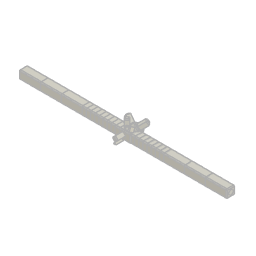
ModularFrame (Autodesk Fusion 360 design; units mm, degrees)
Autodesk Fusion 360 part; units mm, degrees
sketch "Sketch1" plane through (0, 0, 0) normal (0, 0, 1) x (1, 0, 0) in component "BasePart"
  line L0 (5, -5) -> (-5, -5)
  line L1 (-5, -5) -> (-5, 5)
  line L2 (-5, 5) -> (5, 5)
  line L3 (5, 5) -> (5, -5)
  line L4 (5, -5) -> (-5, 5) construction
  line L5 (-5, -5) -> (5, 5) construction
  dimension "drivingDimension" = 10
  constraint horizontal L0
  constraint perpendicular L0 L1
  constraint parallel L0 L2
  constraint parallel L1 L3
  constraint coincident L4 origin
  constraint coincident L5 origin
  constraint equal L1 L2
  measures "drivingDimension" distance of L1.end L2.end
extrude "Extrude1" add sketch "Sketch1" along normal blind 10 makes body 1 in component "BasePart"
chamfer "Chamfer1" distance 1 angle 45 6 faces at (5, 1.6667, 3.3333) (-1.6667, 1.6667, 10) (1.6667, -5, 3.3333) (-5, -1.6667, 3.3333) (-1.6667, 5, 3.3333) (-1.6667, 1.6667, 0) on bodies 1 in component "BasePart"
sketch "Sketch1 (2)" plane through (0, 0, 0) normal (0, 1, 0) x (1, 0, 0) in component "Peg"
  line L0 (0, -3.3333) -> (-3.3333, 0)
  line L1 (-3.3333, 0) -> (0, 3.3333)
  line L2 (0, 3.3333) -> (3.3333, 0)
  line L3 (3.3333, 0) -> (0, -3.3333)
  line L4 (0, 0) -> (3.3333, 0) construction
  line L5 (0, -3.3333) -> (0, 0) construction
  dimension "d266" = 3.3333
  dimension "d267" = 45
  constraint coincident L4.start L5.end
  constraint perpendicular L0 L1
  constraint parallel L0 L2
  constraint parallel L1 L3
  constraint horizontal L4
  constraint vertical L5
  constraint equal L0 L1
  measures "d266" distance of L4.start L2.end
  measures "d267" angle of L3 L4
extrude "Extrude1'" add sketch "Sketch1 (2)" along normal blind 10 separate body makes body 2 in component "Peg"
sketch "Sketch1 (3)" plane through (0, 0, 0) normal (0, 1, 0) x (1, 0, 0) in component "PegHoleCuttingTool"
  line L0 (0, -3.5333) -> (-3.5333, 0)
  line L1 (-3.5333, 0) -> (0, 3.5333)
  line L2 (0, 3.5333) -> (3.5333, 0)
  line L3 (3.5333, 0) -> (0, -3.5333)
  line L4 (0, -3.5333) -> (0, 0) construction
  line L5 (0, 0) -> (3.5333, 0) construction
  dimension "d268" = 3.5333
  dimension "d269" = 45
  constraint coincident L4.end L5.start
  constraint perpendicular L0 L1
  constraint parallel L0 L2
  constraint parallel L1 L3
  constraint vertical L4
  constraint perpendicular L4 L5
  constraint equal L0 L1
  measures "d268" distance of L4.end L2.end
  measures "d269" angle of L3 L5
extrude "Extrude1''" add sketch "Sketch1 (3)" along normal blind 10 separate body makes body 3 in component "PegHoleCuttingTool"
chamfer "Chamfer1'" distance 1 angle 45 1 faces at (0, 10, 1.1111) on bodies 2 in component "Peg"
sketch "Sketch1 (4)" plane through (0, 0, 0) normal (0, 0, 1) x (1, 0, 0) in component "Edge_2x"
  line L0 (10, 5) -> (-10, 5)
  line L1 (-10, 5) -> (-10, -5)
  line L2 (-10, -5) -> (10, -5)
  line L3 (10, -5) -> (10, 5)
  line L4 (10, 5) -> (-10, -5) construction
  line L5 (-10, 5) -> (10, -5) construction
  dimension "d165" = 20
  dimension "d166" = 10
  constraint horizontal L0
  constraint perpendicular L0 L1
  constraint parallel L0 L2
  constraint parallel L1 L3
  constraint coincident L4 origin
  constraint coincident L5 origin
  measures "d165" distance of L1.end L2.end
  measures "d166" distance of L0.end L1.end
extrude "Extrude1'''" add sketch "Sketch1 (4)" along normal blind 10 separate body makes body 4 in component "Edge_2x"
chamfer "Chamfer1''" distance 1 angle 45 6 faces at (-3.3333, -5, 3.3333) (-3.3333, 1.6667, 10) (-10, 1.6667, 3.3333) (3.3333, 5, 3.3333) (10, -1.6667, 3.3333) (-3.3333, 1.6667, 0) on bodies 4 in component "Edge_2x"
combine "Combine1" operation cut target body 4 tool bodies 3 3 body 3 seen with x (0, -1, 0) y (-1, 0, 0) z (0, 0, -1) at (0, 0, 5) body 3 seen with x (0, 1, 0) y (1, 0, 0) z (0, 0, -1) at (0, 0, 5) keep tools in component "Edge_2x"
sketch "Sketch1 (5)" plane through (0, 0, 0) normal (0, 0, 1) x (1, 0, 0) in component "Edge_3x"
  line L0 (15, 5) -> (-15, 5)
  line L1 (-15, 5) -> (-15, -5)
  line L2 (-15, -5) -> (15, -5)
  line L3 (15, -5) -> (15, 5)
  line L4 (15, 5) -> (-15, -5) construction
  line L5 (-15, 5) -> (15, -5) construction
  dimension "d165_1" = 30
  dimension "d166_1" = 10
  constraint horizontal L0
  constraint perpendicular L0 L1
  constraint parallel L0 L2
  constraint parallel L1 L3
  constraint coincident L4 origin
  constraint coincident L5 origin
  measures "d165_1" distance of L1.end L2.end
  measures "d166_1" distance of L0.end L1.end
extrude "Extrude1''''" add sketch "Sketch1 (5)" along normal blind 10 separate body makes body 5 in component "Edge_3x"
chamfer "Chamfer1'''" distance 1 angle 45 6 faces at (-5, -5, 3.3333) (-5, -1.6667, 10) (-15, 1.6667, 3.3333) (5, 5, 3.3333) (15, -1.6667, 3.3333) (-5, -1.6667, 0) on bodies 5 in component "Edge_3x"
sketch "Sketch1 (6)" plane through (0, 0, 0) normal (0, 0, 1) x (1, 0, 0) in component "Edge_4x"
  line L0 (20, 5) -> (-20, 5)
  line L1 (-20, 5) -> (-20, -5)
  line L2 (-20, -5) -> (20, -5)
  line L3 (20, -5) -> (20, 5)
  line L4 (20, 5) -> (-20, -5) construction
  line L5 (-20, 5) -> (20, -5) construction
  dimension "d165_1_1" = 40
  dimension "d166_1_1" = 10
  constraint horizontal L0
  constraint perpendicular L0 L1
  constraint parallel L0 L2
  constraint parallel L1 L3
  constraint coincident L4 origin
  constraint coincident L5 origin
  measures "d165_1_1" distance of L1.end L2.end
  measures "d166_1_1" distance of L0.end L1.end
extrude "Extrude1'''''" add sketch "Sketch1 (6)" along normal blind 10 separate body makes body 6 in component "Edge_4x"
chamfer "Chamfer1''''" distance 1 angle 45 6 faces at (-6.6667, -5, 3.3333) (-6.6667, 1.6667, 10) (-20, 1.6667, 3.3333) (6.6667, 5, 3.3333) (20, -1.6667, 3.3333) (-6.6667, 1.6667, 0) on bodies 6 in component "Edge_4x"
sketch "Sketch1 (7)" plane through (0, 0, 0) normal (0, 0, 1) x (1, 0, 0) in component "Edge_5x"
  line L0 (25, 5) -> (-25, 5)
  line L1 (-25, 5) -> (-25, -5)
  line L2 (-25, -5) -> (25, -5)
  line L3 (25, -5) -> (25, 5)
  line L4 (25, 5) -> (-25, -5) construction
  line L5 (-25, 5) -> (25, -5) construction
  dimension "d165_1_2" = 50
  dimension "d166_1_2" = 10
  constraint horizontal L0
  constraint perpendicular L0 L1
  constraint parallel L0 L2
  constraint parallel L1 L3
  constraint coincident L4 origin
  constraint coincident L5 origin
  measures "d165_1_2" distance of L1.end L2.end
  measures "d166_1_2" distance of L0.end L1.end
extrude "Extrude1''''''" add sketch "Sketch1 (7)" along normal blind 10 separate body makes body 7 in component "Edge_5x"
chamfer "Chamfer1'''''" distance 1 angle 45 6 faces at (-8.3333, -5, 3.3333) (-8.3333, 1.6667, 10) (-25, 1.6667, 3.3333) (8.3333, 5, 3.3333) (25, -1.6667, 3.3333) (-8.3333, 1.6667, 0) on bodies 7 in component "Edge_5x"
sketch "Sketch1 (8)" plane through (0, 0, 0) normal (0, 0, 1) x (1, 0, 0) in component "Edge_6x"
  line L0 (30, 5) -> (-30, 5)
  line L1 (-30, 5) -> (-30, -5)
  line L2 (-30, -5) -> (30, -5)
  line L3 (30, -5) -> (30, 5)
  line L4 (30, 5) -> (-30, -5) construction
  line L5 (-30, 5) -> (30, -5) construction
  dimension "d165_1_3" = 60
  dimension "d166_1_3" = 10
  constraint horizontal L0
  constraint perpendicular L0 L1
  constraint parallel L0 L2
  constraint parallel L1 L3
  constraint coincident L4 origin
  constraint coincident L5 origin
  measures "d165_1_3" distance of L1.end L2.end
  measures "d166_1_3" distance of L0.end L1.end
extrude "Extrude1'''''''" add sketch "Sketch1 (8)" along normal blind 10 separate body makes body 8 in component "Edge_6x"
chamfer "Chamfer1''''''" distance 1 angle 45 6 faces at (-10, -5, 3.3333) (-10, 1.6667, 10) (-30, 1.6667, 3.3333) (10, 5, 3.3333) (30, -1.6667, 3.3333) (-10, 1.6667, 0) on bodies 8 in component "Edge_6x"
sketch "Sketch1 (9)" plane through (0, 0, 0) normal (0, 0, 1) x (1, 0, 0) in component "Edge_7x"
  line L0 (35, 5) -> (-35, 5)
  line L1 (-35, 5) -> (-35, -5)
  line L2 (-35, -5) -> (35, -5)
  line L3 (35, -5) -> (35, 5)
  line L4 (35, 5) -> (-35, -5) construction
  line L5 (-35, 5) -> (35, -5) construction
  dimension "d165_1_4" = 70
  dimension "d166_1_4" = 10
  constraint horizontal L0
  constraint perpendicular L0 L1
  constraint parallel L0 L2
  constraint parallel L1 L3
  constraint coincident L4 origin
  constraint coincident L5 origin
  measures "d165_1_4" distance of L1.end L2.end
  measures "d166_1_4" distance of L0.end L1.end
extrude "Extrude1''''''''" add sketch "Sketch1 (9)" along normal blind 10 separate body makes body 9 in component "Edge_7x"
chamfer "Chamfer1'''''''" distance 1 angle 45 6 faces at (-11.6667, -5, 3.3333) (-11.6667, 1.6667, 10) (-35, 1.6667, 3.3333) (11.6667, 5, 3.3333) (35, -1.6667, 3.3333) (-11.6667, 1.6667, 0) on bodies 9 in component "Edge_7x"
sketch "Sketch1 (10)" plane through (0, 0, 0) normal (0, 0, 1) x (1, 0, 0) in component "Edge_8x"
  line L0 (40, 5) -> (-40, 5)
  line L1 (-40, 5) -> (-40, -5)
  line L2 (-40, -5) -> (40, -5)
  line L3 (40, -5) -> (40, 5)
  line L4 (40, 5) -> (-40, -5) construction
  line L5 (-40, 5) -> (40, -5) construction
  dimension "d165_1_5" = 80
  dimension "d166_1_5" = 10
  constraint horizontal L0
  constraint perpendicular L0 L1
  constraint parallel L0 L2
  constraint parallel L1 L3
  constraint coincident L4 origin
  constraint coincident L5 origin
  measures "d165_1_5" distance of L1.end L2.end
  measures "d166_1_5" distance of L0.end L1.end
extrude "Extrude1'''''''''" add sketch "Sketch1 (10)" along normal blind 10 separate body makes body 10 in component "Edge_8x"
chamfer "Chamfer1''''''''" distance 1 angle 45 6 faces at (-13.3333, -5, 6.6667) (13.3333, 1.6667, 10) (-40, 1.6667, 3.3333) (13.3333, 5, 6.6667) (40, -1.6667, 3.3333) (13.3333, 1.6667, 0) on bodies 10 in component "Edge_8x"
sketch "Sketch1 (11)" plane through (0, 0, 0) normal (0, 0, 1) x (1, 0, 0) in component "Edge_9x"
  line L0 (45, 5) -> (-45, 5)
  line L1 (-45, 5) -> (-45, -5)
  line L2 (-45, -5) -> (45, -5)
  line L3 (45, -5) -> (45, 5)
  line L4 (45, 5) -> (-45, -5) construction
  line L5 (-45, 5) -> (45, -5) construction
  dimension "d165_1_6" = 90
  dimension "d166_1_6" = 10
  constraint horizontal L0
  constraint perpendicular L0 L1
  constraint parallel L0 L2
  constraint parallel L1 L3
  constraint coincident L4 origin
  constraint coincident L5 origin
  measures "d165_1_6" distance of L1.end L2.end
  measures "d166_1_6" distance of L0.end L1.end
extrude "Extrude1''''''''''" add sketch "Sketch1 (11)" along normal blind 10 separate body makes body 11 in component "Edge_9x"
chamfer "Chamfer1'''''''''" distance 1 angle 45 6 faces at (-15, -5, 3.3333) (15, -1.6667, 10) (-45, 1.6667, 3.3333) (15, 5, 3.3333) (45, -1.6667, 3.3333) (15, -1.6667, 0) on bodies 11 in component "Edge_9x"
sketch "Sketch1 (12)" plane through (0, 0, 0) normal (0, 0, 1) x (1, 0, 0) in component "Edge_10x"
  line L0 (50, 5) -> (-50, 5)
  line L1 (-50, 5) -> (-50, -5)
  line L2 (-50, -5) -> (50, -5)
  line L3 (50, -5) -> (50, 5)
  line L4 (50, 5) -> (-50, -5) construction
  line L5 (-50, 5) -> (50, -5) construction
  dimension "d165_1_7" = 100
  dimension "d166_1_7" = 10
  constraint horizontal L0
  constraint perpendicular L0 L1
  constraint parallel L0 L2
  constraint parallel L1 L3
  constraint coincident L4 origin
  constraint coincident L5 origin
  measures "d165_1_7" distance of L1.end L2.end
  measures "d166_1_7" distance of L0.end L1.end
extrude "Extrude1'''''''''''" add sketch "Sketch1 (12)" along normal blind 10 separate body makes body 12 in component "Edge_10x"
chamfer "Chamfer1''''''''''" distance 1 angle 45 6 faces at (-16.6667, -5, 3.3333) (16.6667, -1.6667, 10) (-50, 1.6667, 3.3333) (16.6667, 5, 3.3333) (50, -1.6667, 3.3333) (16.6667, -1.6667, 0) on bodies 12 in component "Edge_10x"
sketch "Sketch1 (13)" plane through (0, 0, 0) normal (0, 0, 1) x (1, 0, 0) in component "Edge_15x"
  line L0 (75, 5) -> (-75, 5)
  line L1 (-75, 5) -> (-75, -5)
  line L2 (-75, -5) -> (75, -5)
  line L3 (75, -5) -> (75, 5)
  line L4 (75, 5) -> (-75, -5) construction
  line L5 (-75, 5) -> (75, -5) construction
  dimension "d165_1_8" = 150
  dimension "d166_1_8" = 10
  constraint horizontal L0
  constraint perpendicular L0 L1
  constraint parallel L0 L2
  constraint parallel L1 L3
  constraint coincident L4 origin
  constraint coincident L5 origin
  measures "d165_1_8" distance of L1.end L2.end
  measures "d166_1_8" distance of L0.end L1.end
extrude "Extrude1''''''''''''" add sketch "Sketch1 (13)" along normal blind 10 separate body makes body 13 in component "Edge_15x"
chamfer "Chamfer1'''''''''''" distance 1 angle 45 6 faces at (-25, -5, 6.6667) (25, -1.6667, 10) (-75, 1.6667, 3.3333) (25, 5, 3.3333) (75, -1.6667, 3.3333) (25, -1.6667, 0) on bodies 13 in component "Edge_15x"
sketch "Sketch1 (14)" plane through (0, 0, 0) normal (0, 0, 1) x (1, 0, 0) in component "Edge_20x"
  line L0 (100, 5) -> (-100, 5)
  line L1 (-100, 5) -> (-100, -5)
  line L2 (-100, -5) -> (100, -5)
  line L3 (100, -5) -> (100, 5)
  line L4 (100, 5) -> (-100, -5) construction
  line L5 (-100, 5) -> (100, -5) construction
  dimension "d165_1_8_1" = 200
  dimension "d166_1_8_1" = 10
  constraint horizontal L0
  constraint perpendicular L0 L1
  constraint parallel L0 L2
  constraint parallel L1 L3
  constraint coincident L4 origin
  constraint coincident L5 origin
  measures "d165_1_8_1" distance of L1.end L2.end
  measures "d166_1_8_1" distance of L0.end L1.end
extrude "Extrude1'''''''''''''" add sketch "Sketch1 (14)" along normal blind 10 separate body makes body 14 in component "Edge_20x"
chamfer "Chamfer1''''''''''''" distance 1 angle 45 6 faces at (-33.3333, -5, 3.3333) (33.3333, 1.6667, 10) (-100, 1.6667, 3.3333) (33.3333, 5, 3.3333) (100, -1.6667, 3.3333) (33.3333, 1.6667, 0) on bodies 14 in component "Edge_20x"
sketch "Sketch1 (15)" plane through (0, 0, 0) normal (0, 0, 1) x (1, 0, 0) in component "Edge_25x"
  line L0 (125, 5) -> (-125, 5)
  line L1 (-125, 5) -> (-125, -5)
  line L2 (-125, -5) -> (125, -5)
  line L3 (125, -5) -> (125, 5)
  line L4 (125, 5) -> (-125, -5) construction
  line L5 (-125, 5) -> (125, -5) construction
  dimension "d165_1_8_2" = 250
  dimension "d166_1_8_2" = 10
  constraint horizontal L0
  constraint perpendicular L0 L1
  constraint parallel L0 L2
  constraint parallel L1 L3
  constraint coincident L4 origin
  constraint coincident L5 origin
  measures "d165_1_8_2" distance of L1.end L2.end
  measures "d166_1_8_2" distance of L0.end L1.end
extrude "Extrude1''''''''''''''" add sketch "Sketch1 (15)" along normal blind 10 separate body makes body 15 in component "Edge_25x"
chamfer "Chamfer1'''''''''''''" distance 1 angle 45 6 faces at (-41.6667, -5, 3.3333) (41.6667, -1.6667, 10) (-125, 1.6667, 3.3333) (41.6667, 5, 3.3333) (125, -1.6667, 3.3333) (41.6667, -1.6667, 0) on bodies 15 in component "Edge_25x"
combine "Combine2" operation cut target body 5 tool bodies 3 3 body 3 seen with x (0, 1, 0) y (-1, 0, 0) z (0, 0, 1) at (15, 0, 5) body 3 seen with x (0, -1, 0) y (1, 0, 0) z (0, 0, 1) at (-15, 0, 5) keep tools in component "Edge_3x"
combine "Combine2'" operation cut target body 6 tool bodies 3 3 body 3 seen with x (0, 1, 0) y (-1, 0, 0) z (0, 0, 1) at (20, 0, 5) body 3 seen with x (0, 0, 1) y (1, 0, 0) z (0, 1, 0) at (-20, 0, 5) keep tools in component "Edge_4x"
combine "Combine2''" operation cut target body 7 tool bodies 3 3 body 3 seen with x (0, 1, 0) y (-1, 0, 0) z (0, 0, 1) at (25, 0, 5) body 3 seen with x (0, -1, 0) y (1, 0, 0) z (0, 0, 1) at (-25, 0, 5) keep tools in component "Edge_5x"
combine "Combine2'''" operation cut target body 8 tool bodies 3 3 body 3 seen with x (0, 1, 0) y (-1, 0, 0) z (0, 0, 1) at (30, 0, 5) body 3 seen with x (0, -1, 0) y (1, 0, 0) z (0, 0, 1) at (-30, 0, 5) keep tools in component "Edge_6x"
combine "Combine2''''" operation cut target body 9 tool bodies 3 3 body 3 seen with x (0, -1, 0) y (1, 0, 0) z (0, 0, 1) at (-35, 0, 5) body 3 seen with x (0, 1, 0) y (-1, 0, 0) z (0, 0, 1) at (35, 0, 5) keep tools in component "Edge_7x"
combine "Combine2'''''" operation cut target body 10 tool bodies 3 3 body 3 seen with x (0, -1, 0) y (1, 0, 0) z (0, 0, 1) at (-40, 0, 5) body 3 seen with x (0, 1, 0) y (-1, 0, 0) z (0, 0, 1) at (40, 0, 5) keep tools in component "Edge_8x"
combine "Combine2''''''" operation cut target body 11 tool bodies 3 3 body 3 seen with x (0, 1, 0) y (-1, 0, 0) z (0, 0, 1) at (45, 0, 5) body 3 seen with x (0, -1, 0) y (1, 0, 0) z (0, 0, 1) at (-45, 0, 5) keep tools in component "Edge_9x"
combine "Combine2'''''''" operation cut target body 12 tool bodies 3 3 body 3 seen with x (0, 1, 0) y (-1, 0, 0) z (0, 0, 1) at (50, 0, 5) body 3 seen with x (0, -1, 0) y (1, 0, 0) z (0, 0, 1) at (-50, 0, 5) keep tools in component "Edge_10x"
combine "Combine2''''''''" operation cut target body 13 tool bodies 3 3 body 3 seen with x (0, -1, 0) y (1, 0, 0) z (0, 0, 1) at (-75, 0, 5) body 3 seen with x (0, 1, 0) y (-1, 0, 0) z (0, 0, 1) at (75, 0, 5) keep tools in component "Edge_15x"
combine "Combine2'''''''''" operation cut target body 14 tool bodies 3 3 body 3 seen with x (0, 1, 0) y (-1, 0, 0) z (0, 0, 1) at (100, 0, 5) body 3 seen with x (0, -1, 0) y (1, 0, 0) z (0, 0, 1) at (-100, 0, 5) keep tools in component "Edge_20x"
combine "Combine2''''''''''" operation cut target body 15 tool bodies 3 3 body 3 seen with x (0, 1, 0) y (-1, 0, 0) z (0, 0, 1) at (125, 0, 5) body 3 seen with x (0, -1, 0) y (1, 0, 0) z (0, 0, 1) at (-125, 0, 5) keep tools in component "Edge_25x"
sketch "Sketch1 (16)" plane through (0, 0, 0) normal (1, 0, 0) x (0, 1, 0) in component "Support"
  line L0 (0, 0) -> (3.3333, 0)
  line L1 (1.6667, 0) -> (1.6667, 1.6667) construction
  line L2 (1.6667, 1.6667) -> (3.3333, 0)
  line L3 (0, 0) -> (1.6667, 1.6667)
  dimension "d272" = 3.3333
  dimension "d273" = 1.6667
  constraint coincident L0.start L3.start
  constraint horizontal L0
  constraint midpoint L0 L1.start
  constraint perpendicular L0 L1
  measures "d272" distance of L0.start L0.end
  measures "d273" distance of L1.start L1.end
extrude "Extrude1'''''''''''''''" add sketch "Sketch1 (16)" along normal blind 9 separate body makes body 16 in component "Support"
combine "Combine1'" operation add target body 1 tool bodies 2 2 2 2 2 2 body 2 seen with x (0, 1, 0) y (-1, 0, 0) z (0, 0, 1) at (-5, 0, 5) body 2 seen with x (1, 0, 0) y (0, 0, 1) z (0, -1, 0) at (0, 0, 10) body 2 seen with x (1, 0, 0) y (0, 0, -1) z (0, 1, 0) at (0, 0, 0) body 2 seen with x (1, 0, 0) y (0, -1, 0) z (0, 0, -1) at (0, -5, 5) body 2 seen with x (1, 0, 0) y (0, 1, 0) z (0, 0, 1) at (0, 5, 5) body 2 seen with x (0, -1, 0) y (1, 0, 0) z (0, 0, 1) at (5, 0, 5) keep tools result as body 17 in component "AsNewCombinedComponent"
move_body "Align2" bodies 17 to x (0.788675, -0.211325, -0.57735) y (-0.211325, 0.788675, -0.57735) z (0.57735, 0.57735, 0.57735) at (1.4161, 1.4161, 4.6188) in component "AsNewCombinedComponent"
move_body "Move2" bodies 4 to x (1, 0, 0) y (0, 1, 0) z (0, 0, 1) at (170, -150, 0) in component "Edge_2x"
component "BasePart" placed x (1, 0, 0) y (0, 1, 0) z (0, 0, 1) at (0, 0, 0)
component "Peg" placed x (1, 0, 0) y (0, 1, 0) z (0, 0, 1) at (0, 0, 0)
component "PegHoleCuttingTool" placed x (1, 0, 0) y (0, 1, 0) z (0, 0, 1) at (0, 0, 0)
component "Support" placed x (0, -1, 0) y (1, 0, 0) z (0, 0, 1) at (-1.6667, -5, 0)
component "Connector_Extender" placed x (1, 0, 0) y (0, 1, 0) z (0, 0, 1) at (0, 0, 0)
component "Connector_3-sided_flat" placed x (1, 0, 0) y (0, 1, 0) z (0, 0, 1) at (0, 0, 0)
component "Connector_3-sided_corner" placed x (1, 0, 0) y (0, 1, 0) z (0, 0, 1) at (0, 0, 0)
component "Connector_4-sided_flat" placed x (1, 0, 0) y (0, 1, 0) z (0, 0, 1) at (0, 0, 0)
component "Connector_4-sided_corner" placed x (1, 0, 0) y (0, 1, 0) z (0, 0, 1) at (0, 0, 0)
component "Connector_5-sided" placed x (1, 0, 0) y (0, 1, 0) z (0, 0, 1) at (0, 0, 0)
component "Connector_6-sided" placed x (1, 0, 0) y (0, 1, 0) z (0, 0, 1) at (0, 0, 0)
component "Edge_2x" placed x (1, 0, 0) y (0, 1, 0) z (0, 0, 1) at (0, 0, 0)
component "Edge_3x" placed x (1, 0, 0) y (0, 1, 0) z (0, 0, 1) at (0, 0, 0)
component "Edge_4x" placed x (1, 0, 0) y (0, 1, 0) z (0, 0, 1) at (0, 0, 0)
component "Edge_5x" placed x (1, 0, 0) y (0, 1, 0) z (0, 0, 1) at (0, 0, 0)
component "Edge_6x" placed x (1, 0, 0) y (0, 1, 0) z (0, 0, 1) at (0, 0, 0)
component "Edge_7x" placed x (1, 0, 0) y (0, 1, 0) z (0, 0, 1) at (0, 0, 0)
component "Edge_8x" placed x (1, 0, 0) y (0, 1, 0) z (0, 0, 1) at (0, 0, 0)
component "Edge_9x" placed x (1, 0, 0) y (0, 1, 0) z (0, 0, 1) at (0, 0, 0)
component "Edge_10x" placed x (1, 0, 0) y (0, 1, 0) z (0, 0, 1) at (0, 0, 0)
component "Edge_15x" placed x (1, 0, 0) y (0, 1, 0) z (0, 0, 1) at (0, 0, 0)
component "Edge_20x" placed x (1, 0, 0) y (0, 1, 0) z (0, 0, 1) at (0, 0, 0)
component "Edge_25x" placed x (1, 0, 0) y (0, 1, 0) z (0, 0, 1) at (0, 0, 0)
component "ElementsShowcase" placed x (1, 0, 0) y (0, 1, 0) z (0, 0, 1) at (0, 0, 0)
component "BasePart" placed x (1, 0, 0) y (0, 1, 0) z (0, 0, 1) at (0, 0, 0) in component "Connector_Extender"
component "Peg" placed x (1, 0, 0) y (0, 1, 0) z (0, 0, 1) at (0, 5, 5) in component "Connector_Extender"
component "Peg" placed x (1, 0, 0) y (0, -1, 0) z (0, 0, -1) at (0, -5, 5) in component "Connector_Extender"
component "Support" placed x (0, 1, 0) y (-1, 0, 0) z (0, 0, 1) at (1.6667, 6, 0) in component "Connector_Extender"
component "Support" placed x (0, -1, 0) y (1, 0, 0) z (0, 0, 1) at (-1.6667, -6, 0) in component "Connector_Extender"
component "BasePart" placed x (1, 0, 0) y (0, 1, 0) z (0, 0, 1) at (0, 0, 0) in component "Connector_3-sided_flat"
component "Peg" placed x (1, 0, 0) y (0, 1, 0) z (0, 0, 1) at (0, 5, 5) in component "Connector_3-sided_flat"
component "Peg" placed x (0, -1, 0) y (1, 0, 0) z (0, 0, 1) at (5, 0, 5) in component "Connector_3-sided_flat"
component "Peg" placed x (1, 0, 0) y (0, -1, 0) z (0, 0, -1) at (0, -5, 5) in component "Connector_3-sided_flat"
component "Support" placed x (0, -1, 0) y (1, 0, 0) z (0, 0, 1) at (-1.6667, -6, 0) in component "Connector_3-sided_flat"
component "Support" placed x (0, 1, 0) y (-1, 0, 0) z (0, 0, 1) at (1.6667, 6, 0) in component "Connector_3-sided_flat"
component "Support" placed x (1, 0, 0) y (0, 1, 0) z (0, 0, 1) at (6, -1.6667, 0) in component "Connector_3-sided_flat"
component "BasePart" placed x (1, 0, 0) y (0, 1, 0) z (0, 0, 1) at (0, 0, 0) in component "Connector_3-sided_corner"
component "Peg" placed x (1, 0, 0) y (0, -1, 0) z (0, 0, -1) at (0, -5, 5) in component "Connector_3-sided_corner"
component "Peg" placed x (1, 0, 0) y (0, 0, 1) z (0, -1, 0) at (0, 0, 10) in component "Connector_3-sided_corner"
component "Peg" placed x (0, -1, 0) y (1, 0, 0) z (0, 0, 1) at (5, 0, 5) in component "Connector_3-sided_corner"
component "Support" placed x (0, -1, 0) y (1, 0, 0) z (0, 0, 1) at (-1.6667, -6, 0) in component "Connector_3-sided_corner"
component "Support" placed x (1, 0, 0) y (0, 1, 0) z (0, 0, 1) at (6, -1.6667, 0) in component "Connector_3-sided_corner"
component "BasePart" placed x (1, 0, 0) y (0, 1, 0) z (0, 0, 1) at (0, 0, 0) in component "Connector_4-sided_flat"
component "Peg" placed x (1, 0, 0) y (0, 1, 0) z (0, 0, 1) at (0, 5, 5) in component "Connector_4-sided_flat"
component "Peg" placed x (0, 1, 0) y (-1, 0, 0) z (0, 0, 1) at (-5, 0, 5) in component "Connector_4-sided_flat"
component "Peg" placed x (0, -1, 0) y (1, 0, 0) z (0, 0, 1) at (5, 0, 5) in component "Connector_4-sided_flat"
component "Peg" placed x (1, 0, 0) y (0, -1, 0) z (0, 0, -1) at (0, -5, 5) in component "Connector_4-sided_flat"
component "Support" placed x (0, -1, 0) y (1, 0, 0) z (0, 0, 1) at (-1.6667, -6, 0) in component "Connector_4-sided_flat"
component "Support" placed x (-1, 0, 0) y (0, -1, 0) z (0, 0, 1) at (-6, 1.6667, 0) in component "Connector_4-sided_flat"
component "Support" placed x (1, 0, 0) y (0, 1, 0) z (0, 0, 1) at (6, -1.6667, 0) in component "Connector_4-sided_flat"
component "Support" placed x (0, 1, 0) y (-1, 0, 0) z (0, 0, 1) at (1.6667, 6, 0) in component "Connector_4-sided_flat"
component "BasePart" placed x (1, 0, 0) y (0, 1, 0) z (0, 0, 1) at (0, 0, 0) in component "Connector_4-sided_corner"
component "Peg" placed x (0, -1, 0) y (1, 0, 0) z (0, 0, 1) at (5, 0, 5) in component "Connector_4-sided_corner"
component "Peg" placed x (1, 0, 0) y (0, 0, 1) z (0, -1, 0) at (0, 0, 10) in component "Connector_4-sided_corner"
component "Peg" placed x (1, 0, 0) y (0, 1, 0) z (0, 0, 1) at (0, 5, 5) in component "Connector_4-sided_corner"
component "Peg" placed x (1, 0, 0) y (0, -1, 0) z (0, 0, -1) at (0, -5, 5) in component "Connector_4-sided_corner"
component "Support" placed x (0, 1, 0) y (-1, 0, 0) z (0, 0, 1) at (1.6667, 6, 0) in component "Connector_4-sided_corner"
component "Support" placed x (1, 0, 0) y (0, 1, 0) z (0, 0, 1) at (6, -1.6667, 0) in component "Connector_4-sided_corner"
component "Support" placed x (0, -1, 0) y (1, 0, 0) z (0, 0, 1) at (-1.6667, -6, 0) in component "Connector_4-sided_corner"
component "BasePart" placed x (1, 0, 0) y (0, 1, 0) z (0, 0, 1) at (0, 0, 0) in component "Connector_5-sided"
component "Peg" placed x (1, 0, 0) y (0, -1, 0) z (0, 0, -1) at (0, -5, 5) in component "Connector_5-sided"
component "Peg" placed x (0, 1, 0) y (-1, 0, 0) z (0, 0, 1) at (-5, 0, 5) in component "Connector_5-sided"
component "Peg" placed x (1, 0, 0) y (0, 0, 1) z (0, -1, 0) at (0, 0, 10) in component "Connector_5-sided"
component "Peg" placed x (1, 0, 0) y (0, 1, 0) z (0, 0, 1) at (0, 5, 5) in component "Connector_5-sided"
component "Peg" placed x (0, -1, 0) y (1, 0, 0) z (0, 0, 1) at (5, 0, 5) in component "Connector_5-sided"
component "Support" placed x (1, 0, 0) y (0, 1, 0) z (0, 0, 1) at (6, -1.6667, 0) in component "Connector_5-sided"
component "Support" placed x (0, -1, 0) y (1, 0, 0) z (0, 0, 1) at (-1.6667, -6, 0) in component "Connector_5-sided"
component "Support" placed x (0, 1, 0) y (-1, 0, 0) z (0, 0, 1) at (1.6667, 6, 0) in component "Connector_5-sided"
component "Support" placed x (-1, 0, 0) y (0, -1, 0) z (0, 0, 1) at (-6, 1.6667, 0) in component "Connector_5-sided"
component "BasePart" placed x (1, 0, 0) y (0, 1, 0) z (0, 0, 1) at (0, 0, 0) in component "Connector_6-sided"
component "Peg" placed x (0, 1, 0) y (-1, 0, 0) z (0, 0, 1) at (-5, 0, 5) in component "Connector_6-sided"
component "Peg" placed x (1, 0, 0) y (0, 0, 1) z (0, -1, 0) at (0, 0, 10) in component "Connector_6-sided"
component "Peg" placed x (0, -1, 0) y (1, 0, 0) z (0, 0, 1) at (5, 0, 5) in component "Connector_6-sided"
component "Peg" placed x (1, 0, 0) y (0, 1, 0) z (0, 0, 1) at (0, 5, 5) in component "Connector_6-sided"
component "Peg" placed x (1, 0, 0) y (0, 0, -1) z (0, 1, 0) at (0, 0, 0) in component "Connector_6-sided"
component "Peg" placed x (1, 0, 0) y (0, -1, 0) z (0, 0, -1) at (0, -5, 5) in component "Connector_6-sided"
component "AsNewCombinedComponent" placed x (1, 0, 0) y (0, 1, 0) z (0, 0, 1) at (0, 0, 0) in component "Connector_6-sided"
component "PegHoleCuttingTool" placed x (0, -1, 0) y (-1, 0, 0) z (0, 0, -1) at (0, 0, 5) in component "Edge_2x"
component "PegHoleCuttingTool" placed x (0, 1, 0) y (1, 0, 0) z (0, 0, -1) at (0, 0, 5) in component "Edge_2x"
component "PegHoleCuttingTool" placed x (0, 1, 0) y (-1, 0, 0) z (0, 0, 1) at (15, 0, 5) in component "Edge_3x"
component "PegHoleCuttingTool" placed x (0, -1, 0) y (1, 0, 0) z (0, 0, 1) at (-15, 0, 5) in component "Edge_3x"
component "PegHoleCuttingTool" placed x (0, 0, 1) y (1, 0, 0) z (0, 1, 0) at (-20, 0, 5) in component "Edge_4x"
component "PegHoleCuttingTool" placed x (0, 1, 0) y (-1, 0, 0) z (0, 0, 1) at (20, 0, 5) in component "Edge_4x"
component "PegHoleCuttingTool" placed x (0, 1, 0) y (-1, 0, 0) z (0, 0, 1) at (25, 0, 5) in component "Edge_5x"
component "PegHoleCuttingTool" placed x (0, -1, 0) y (1, 0, 0) z (0, 0, 1) at (-25, 0, 5) in component "Edge_5x"
component "PegHoleCuttingTool" placed x (0, -1, 0) y (1, 0, 0) z (0, 0, 1) at (-30, 0, 5) in component "Edge_6x"
component "PegHoleCuttingTool" placed x (0, 1, 0) y (-1, 0, 0) z (0, 0, 1) at (30, 0, 5) in component "Edge_6x"
component "PegHoleCuttingTool" placed x (0, -1, 0) y (1, 0, 0) z (0, 0, 1) at (-35, 0, 5) in component "Edge_7x"
component "PegHoleCuttingTool" placed x (0, 1, 0) y (-1, 0, 0) z (0, 0, 1) at (35, 0, 5) in component "Edge_7x"
component "PegHoleCuttingTool" placed x (0, -1, 0) y (1, 0, 0) z (0, 0, 1) at (-40, 0, 5) in component "Edge_8x"
component "PegHoleCuttingTool" placed x (0, 1, 0) y (-1, 0, 0) z (0, 0, 1) at (40, 0, 5) in component "Edge_8x"
component "PegHoleCuttingTool" placed x (0, -1, 0) y (1, 0, 0) z (0, 0, 1) at (-45, 0, 5) in component "Edge_9x"
component "PegHoleCuttingTool" placed x (0, 1, 0) y (-1, 0, 0) z (0, 0, 1) at (45, 0, 5) in component "Edge_9x"
component "PegHoleCuttingTool" placed x (0, 1, 0) y (-1, 0, 0) z (0, 0, 1) at (50, 0, 5) in component "Edge_10x"
component "PegHoleCuttingTool" placed x (0, -1, 0) y (1, 0, 0) z (0, 0, 1) at (-50, 0, 5) in component "Edge_10x"
component "PegHoleCuttingTool" placed x (0, 1, 0) y (-1, 0, 0) z (0, 0, 1) at (75, 0, 5) in component "Edge_15x"
component "PegHoleCuttingTool" placed x (0, -1, 0) y (1, 0, 0) z (0, 0, 1) at (-75, 0, 5) in component "Edge_15x"
component "PegHoleCuttingTool" placed x (0, -1, 0) y (1, 0, 0) z (0, 0, 1) at (-100, 0, 5) in component "Edge_20x"
component "PegHoleCuttingTool" placed x (0, 1, 0) y (-1, 0, 0) z (0, 0, 1) at (100, 0, 5) in component "Edge_20x"
component "PegHoleCuttingTool" placed x (0, 1, 0) y (-1, 0, 0) z (0, 0, 1) at (125, 0, 5) in component "Edge_25x"
component "PegHoleCuttingTool" placed x (0, -1, 0) y (1, 0, 0) z (0, 0, 1) at (-125, 0, 5) in component "Edge_25x"
component "Connector_Extender" placed x (1, 0, 0) y (0, 1, 0) z (0, 0, 1) at (0, 0, 0) in component "ElementsShowcase"
component "Edge_8x" placed x (1, 0, 0) y (0, 1, 0) z (0, 0, 1) at (0, 0, 0) in component "ElementsShowcase"
component "Edge_9x" placed x (1, 0, 0) y (0, 1, 0) z (0, 0, 1) at (0, 0, 0) in component "ElementsShowcase"
component "Edge_10x" placed x (1, 0, 0) y (0, 1, 0) z (0, 0, 1) at (0, 0, 0) in component "ElementsShowcase"
component "Edge_15x" placed x (1, 0, 0) y (0, 1, 0) z (0, 0, 1) at (0, 0, 0) in component "ElementsShowcase"
component "Edge_20x" placed x (1, 0, 0) y (0, 1, 0) z (0, 0, 1) at (0, 0, 0) in component "ElementsShowcase"
component "Edge_25x" placed x (1, 0, 0) y (0, 1, 0) z (0, 0, 1) at (0, 0, 0) in component "ElementsShowcase"
component "Edge_2x" placed x (1, 0, 0) y (0, 1, 0) z (0, 0, 1) at (0, 0, 0) in component "ElementsShowcase"
component "Edge_5x" placed x (1, 0, 0) y (0, 1, 0) z (0, 0, 1) at (0, 0, 0) in component "ElementsShowcase"
component "Edge_4x" placed x (1, 0, 0) y (0, 1, 0) z (0, 0, 1) at (0, 0, 0) in component "ElementsShowcase"
component "Edge_3x" placed x (1, 0, 0) y (0, 1, 0) z (0, 0, 1) at (0, 0, 0) in component "ElementsShowcase"
component "Edge_6x" placed x (1, 0, 0) y (0, 1, 0) z (0, 0, 1) at (0, 0, 0) in component "ElementsShowcase"
component "Edge_7x" placed x (1, 0, 0) y (0, 1, 0) z (0, 0, 1) at (0, 0, 0) in component "ElementsShowcase"
component "Connector_3-sided_flat" placed x (1, 0, 0) y (0, 1, 0) z (0, 0, 1) at (0, 0, 0) in component "ElementsShowcase"
component "Connector_3-sided_corner" placed x (1, 0, 0) y (0, 1, 0) z (0, 0, 1) at (0, 0, 0) in component "ElementsShowcase"
component "Connector_4-sided_flat" placed x (1, 0, 0) y (0, 1, 0) z (0, 0, 1) at (0, 0, 0) in component "ElementsShowcase"
component "Connector_4-sided_corner" placed x (1, 0, 0) y (0, 1, 0) z (0, 0, 1) at (0, 0, 0) in component "ElementsShowcase"
component "Connector_5-sided" placed x (1, 0, 0) y (0, 1, 0) z (0, 0, 1) at (0, 0, 0) in component "ElementsShowcase"
component "Connector_6-sided" placed x (1, 0, 0) y (0, 1, 0) z (0, 0, 1) at (0, 0, 0) in component "ElementsShowcase"
equation "drivingDimension = DrivingDimension"
equation "d2 = DrivingDimension"
equation "d4 = Chamfer"
equation "pegLength = PegLength"
equation "d9 = Chamfer"
equation "pegLength_1 = PegLength"
equation "drivingDimension_1 = 10 mm"
equation "pegLength_2 = drivingDimension_1"
equation "DrivingDimension = 10 mm"
equation "PegLength = DrivingDimension"
equation "PegWidth = DrivingDimension / 3"
equation "PegCutToolWidth = PegWidth + 0.2 mm"
equation "Chamfer = DrivingDimension / 10"
equation "d165 = DrivingDimension * 2"
equation "d166 = DrivingDimension"
equation "d167 = DrivingDimension"
equation "d169 = Chamfer"
equation "d165_1 = DrivingDimension * 3"
equation "d166_1 = DrivingDimension"
equation "d167_1 = DrivingDimension"
equation "d169_1 = Chamfer"
equation "d165_1_1 = DrivingDimension * 4"
equation "d166_1_1 = DrivingDimension"
equation "d167_1_1 = DrivingDimension"
equation "d169_1_1 = Chamfer"
equation "d165_1_2 = DrivingDimension * 5"
equation "d166_1_2 = DrivingDimension"
equation "d167_1_2 = DrivingDimension"
equation "d169_1_2 = Chamfer"
equation "d165_1_3 = DrivingDimension * 6"
equation "d166_1_3 = DrivingDimension"
equation "d167_1_3 = DrivingDimension"
equation "d169_1_3 = Chamfer"
equation "d165_1_4 = DrivingDimension * 7"
equation "d166_1_4 = DrivingDimension"
equation "d167_1_4 = DrivingDimension"
equation "d169_1_4 = Chamfer"
equation "d165_1_5 = DrivingDimension * 8"
equation "d166_1_5 = DrivingDimension"
equation "d167_1_5 = DrivingDimension"
equation "d169_1_5 = Chamfer"
equation "d165_1_6 = DrivingDimension * 9"
equation "d166_1_6 = DrivingDimension"
equation "d167_1_6 = DrivingDimension"
equation "d169_1_6 = Chamfer"
equation "d165_1_7 = DrivingDimension * 10"
equation "d166_1_7 = DrivingDimension"
equation "d167_1_7 = DrivingDimension"
equation "d169_1_7 = Chamfer"
equation "d165_1_8 = DrivingDimension * 15"
equation "d166_1_8 = DrivingDimension"
equation "d167_1_8 = DrivingDimension"
equation "d169_1_8 = Chamfer"
equation "d165_1_8_1 = DrivingDimension * 20"
equation "d166_1_8_1 = DrivingDimension"
equation "d167_1_8_1 = DrivingDimension"
equation "d169_1_8_1 = Chamfer"
equation "d165_1_8_2 = DrivingDimension * 25"
equation "d166_1_8_2 = DrivingDimension"
equation "d167_1_8_2 = DrivingDimension"
equation "d169_1_8_2 = Chamfer"
equation "d266 = PegWidth"
equation "d268 = PegCutToolWidth"
equation "PegSupportBaseWidth = PegWidth"
equation "PegSupportHeight = DrivingDimension / 2 - PegWidth"
equation "d272 = PegSupportBaseWidth"
equation "d273 = PegSupportHeight"
equation "d274 = PegLength - 1 mm"
